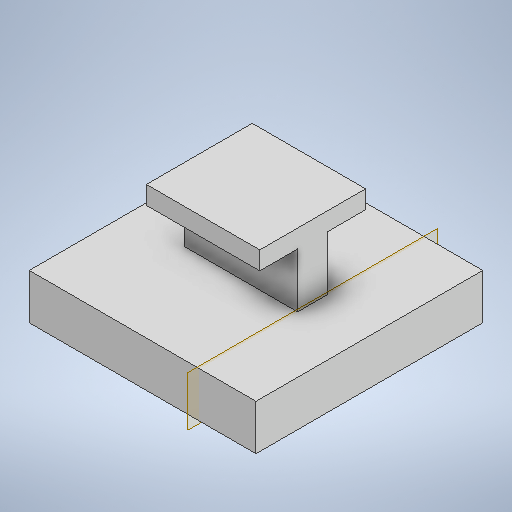
# Autodesk Inventor part: SlangHållareFot
Saved by Autodesk Inventor 2025.2 (Build 292293000, 293)
## iProperties
Created: 2025-01-29
Part Number: SlangHållareFot
Material: Generic
Document SubType Name: Modeling
Designer: 24oscnor
Density: 1 g/cm^3
Appearance: Default
Author: 24oscnor
Autodesk Inventor part; units mm, degrees
ref_plane "YZ Plane" through (0, 0, 0) normal (1, 0, 0) x (0, 1, 0)
ref_plane "XZ Plane" through (0, 0, 0) normal (0, 1, 0) x (-1, 0, 0)
ref_plane "XY Plane" through (0, 0, 0) normal (0, 0, 1) x (1, 0, 0)
sketch "Sketch1" plane through (0, 0, 0) normal (0, 1, 0) x (-1, 0, 0)
  line L0 (0, 0) -> (15, 0)
  line L1 (15, 0) -> (15, 15)
  line L2 (15, 15) -> (0, 15)
  line L3 (0, 15) -> (0, 0)
  dimension "d0" = 15
  dimension "d1" = 15
  constraints: 8 end point, 2 parallel, 1 horizontal, 1 perpendicular
  measures "d0" distance of L0.start L0.end
  measures "d1" distance of L2.end L0.start
extrude "Extrusion1" add sketch "Sketch1" along normal blind 3
ref_plane "Work Plane1" through (-3.75, 0, 15) normal (1, 0, 0) x (0, 0, -1)
sketch "Sketch2" plane through (-3.75, 0, 15) normal (1, 0, 0) x (0, 0, -1)
  line L0 (15, 3) -> (0, 3) projected
  line L1 (9.0593, 3) -> (5.9407, 3)
  line L2 (7.5, 3) -> (7.5, 8.2025)
  line L3 (0, 0) -> (0, 3) projected
  line L4 (7.5, 3) -> (8.5, 3)
  line L5 (8.5, 3) -> (8.5, 7.8)
  line L6 (8.5, 7.8) -> (7.5, 7.8)
  line L7 (7.5, 7.8) -> (7.5, 3)
  line L8 (8.5, 7.8) -> (11, 7.8)
  line L9 (11, 7.8) -> (11, 6.6)
  line L10 (11, 6.6) -> (8.5, 6.6)
  line L11 (8.5, 6.6) -> (8.5, 7.8)
  line L12 (6.5, 3) -> (6.5, 7.8)
  line L13 (6.5, 7.8) -> (7.5, 7.8)
  line L14 (6.5, 7.8) -> (4, 7.8)
  line L15 (4, 7.8) -> (4, 6.6)
  line L16 (4, 6.6) -> (6.5, 6.6)
  line L17 (6.5, 6.6) -> (6.5, 7.8)
  point P0 (15, 0)
  point P1 (6.5, 3)
  point P2 (8.5, 3)
  dimension "d5" = 5.2025
  dimension "d6" = 7.5
  dimension "d7" = 4.8
  dimension "d8" = 1
  dimension "d9" = 7
  dimension "d10" = 1.2
  constraints: 32 end point, 5 symmetric about line, 4 parallel, 3 horizontal, 2 perpendicular, 1 midpoint, 1 point on line, 1 vertical
  measures "d5" distance of L2.start L2.end
  measures "d6" distance between parallel lines of L3 L2
  measures "d7" distance of L4.end L5.end
  measures "d8" distance of L5.end L6.end
  measures "d9" diameter of L9 L2
  measures "d10" distance between parallel lines of L8 L10
extrude "Extrusion2" add sketch "Sketch2" against normal blind 7.5
body "Solid1"
